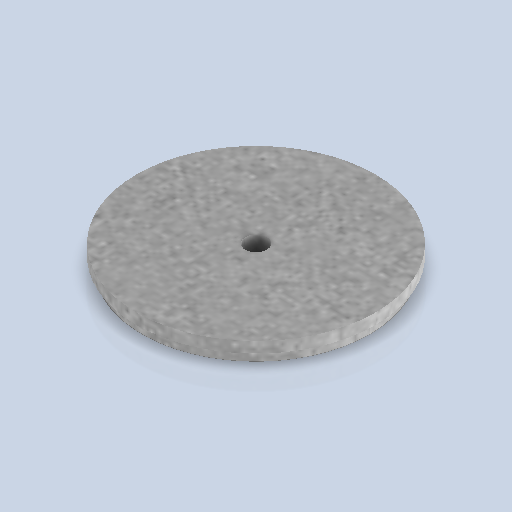
# Autodesk Inventor part: cylinder_cover_top
Saved by Autodesk Inventor 2024.2 (Build 282272000, 272)
## iProperties
Created: 2024-05-05
Part Number: cylinder_cover_top
Material: Glasfaserbeton
Document SubType Name: Modeling
Designer: Fabri
Density: 1.7 g/cm^3
Appearance: Flach - Poliert Grau
Author: Fabri
Autodesk Inventor part; units mm, degrees
ref_plane "YZ Plane" through (0, 0, 0) normal (1, 0, 0) x (0, 1, 0)
ref_plane "XZ Plane" through (0, 0, 0) normal (0, 1, 0) x (-1, 0, 0)
ref_plane "XY Plane" through (0, 0, 0) normal (0, 0, 1) x (1, 0, 0)
sketch "Skizze1" plane through (0, 0, 0) normal (0, 1, 0) x (-1, 0, 0)
  line L0 (0, 0) -> (33, 0)
  line L1 (33, 0) -> (33, -3)
  line L2 (33, -3) -> (31.5, -3)
  line L3 (31.5, -3) -> (31.5, -6)
  line L4 (31.5, -6) -> (0, -6)
  line L5 (0, -6) -> (0, 0)
  dimension "d0" = 3
  dimension "d1" = 3
  dimension "d2" = 63
  dimension "d3" = 66
  constraints: 12 end point, 5 perpendicular, 1 horizontal
  measures "d0" distance between parallel lines of L2 L0
  measures "d1" distance between parallel lines of L4 L2
  measures "d2" diameter of L3 L5
  measures "d3" diameter of L1 L5
revolve "Umdrehung1" add sketch "Skizze1" angle 360 about axis through (0, 0, -6) along (0, 0, 1)
sketch "Skizze2" plane through (0, 0, 0) normal (0, 0, 1) x (1, 0, 0)
  circle A0 centre (0, 0) radius 3
  dimension "d5" = 6
  constraints: 1 centre point, 1 coincident
  measures "d5" diameter of A0
extrude "Extrusion1" cut sketch "Skizze2" against normal up to surface (6 mm away)
equation "\"d1\" = d0"
